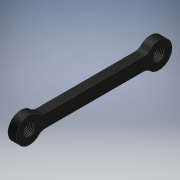
# Autodesk Inventor part: Backplane_Nut
Saved by Autodesk Inventor 2018 (Build 220112000, 112)
## iProperties
Created: 2018-07-04
Part Number: Backplane_Nut
Material: Aluminum 6061
Document SubType Name: Modeling
Designer: Bradley
Density: 2.7 g/cm^3
Appearance: Anodized - Dark Gray
Mass: 0.642644 g
Surface Area: 4.31902 cm^2
Volume: 0.238016 cm^3
Author: Bradley
Autodesk Inventor part; units mm, degrees
ref_plane "YZ Plane" through (0, 0, 0) normal (1, 0, 0) x (0, 1, 0)
ref_plane "XZ Plane" through (0, 0, 0) normal (0, 1, 0) x (-1, 0, 0)
ref_plane "XY Plane" through (0, 0, 0) normal (0, 0, 1) x (1, 0, 0)
sketch "Sketch1" plane through (0, 0, 0) normal (1, 0, 0) x (0, 1, 0)
  line L0 (-15, 0) -> (15, 0) construction
  circle A0 centre (-15, 0) radius 3
  circle A1 centre (15, 0) radius 3
  line L1 (-12.4019, 1.5) -> (12.4019, 1.5)
  line L2 (12.4019, -1.5) -> (-12.4019, -1.5)
  point P0 (0, 0)
  point P1 (0, 0)
  dimension "d0" = 30
  dimension "d1" = 6
  dimension "d2" = 3
  constraints: 6 end point, 4 point on circle, 3 coincident, 2 centre point, 2 horizontal, 2 parallel, 1 equal radius, 1 midpoint
  measures "d0" distance of L0.start L0.end
  measures "d1" diameter of A0
  measures "d2" distance between parallel lines of L2 L1
extrude "Extrusion1" add sketch "Sketch1" along normal mid plane 2
fillet "Fillet1" radius 2 4 edges at (0, -12.4019, 1.5) (0, -12.4019, -1.5) (0, 12.4019, -1.5) (0, 12.4019, 1.5)
sketch "Sketch2" plane through (1, 0, 0) normal (1, 0, 0) x (0, 0, -1)
  arc A0 (-2.1, -12.8576) -> (2.1, -12.8576) centre (0, -15) ccw projected
  arc A1 (1.5, -11.4293) -> (2.1, -12.8576) centre (3.5, -11.4293) ccw projected
  line L0 (1.5, -11.4293) -> (1.5, 11.4293) projected
  arc A2 (2.1, 12.8576) -> (1.5, 11.4293) centre (3.5, 11.4293) ccw projected
  arc A3 (2.1, 12.8576) -> (-2.1, 12.8576) centre (0, 15) ccw projected
  arc A4 (-1.5, 11.4293) -> (-2.1, 12.8576) centre (-3.5, 11.4293) ccw projected
  line L1 (-1.5, 11.4293) -> (-1.5, -11.4293) projected
  arc A5 (-2.1, -12.8576) -> (-1.5, -11.4293) centre (-3.5, -11.4293) ccw projected
  point P0 (0, 0)
  constraints: 2 coincident
hole "Hole1" at (1, -15, 0) at (1, 15, 0) direction (-1, 0, 0) diameter 2.621 end through all thread size "M3x0.35" class "6H" standard "ANSI Metric M Profile"
body "Solid1"
